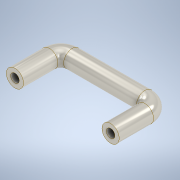
# Autodesk Inventor part: Gagang
Saved by Autodesk Inventor 2021 (Build 250183000, 183)
## iProperties
Created: 2023-04-06
Part Number: Gagang
Material: Generic
Document SubType Name: Modeling
Designer: EF0481
Density: 1 g/cm^3
Appearance: Titanium
Author: EF0481
Autodesk Inventor part; units mm, degrees
ref_plane "YZ Plane" through (0, 0, 0) normal (1, 0, 0) x (0, 1, 0)
ref_plane "XZ Plane" through (0, 0, 0) normal (0, 1, 0) x (-1, 0, 0)
ref_plane "XY Plane" through (0, 0, 0) normal (0, 0, 1) x (1, 0, 0)
sketch "Sketch1" plane through (0, 0, 0) normal (0, 0, 1) x (1, 0, 0)
  circle A0 centre (0, 0) radius 1.5
  circle A1 centre (0, 0) radius 0.75
  dimension "d4" = 3
  dimension "d5" = 1.5
  constraints: 2 centre point, 1 coincident
  measures "d4" diameter of A0
  measures "d5" diameter of A1
sketch3d "3D Sketch1"
  line L0 (0, 0, 0) -> (0, 0, -6)
  arc A0 (0, 0, -6) -> (2, 0, -8) centre (2, 0, -6) ccw
  line L1 (2, 0, -8) -> (14.68, 0, -8)
  arc A1 (14.68, 0, -8) -> (16.68, 0, -6) centre (14.68, 0, -6) ccw
  line L2 (16.68, 0, -6) -> (16.68, 0, 0)
  dimension "d6" = 8
  dimension "d7" = 16.68
  dimension "d8" = 8
  dimension "d9" = 2
  dimension "d10" = 2
sweep "Sweep1" add profiles "Sketch1" path "3D Sketch1"
body "Solid1"
